Autodesk Fusion 360 part; units mm, degrees
note: some values were not read from the file. Set by a fixed rule: which face or edge a step refers to.
(part 2 of 3)
sketch "Sketch11" plane through (87.5, 0, 0) normal (1, 0, 0) x (0, 1, 0)
  arc A0 (-40.5, 50) -> (-42.5, 48) centre (-40.5, 48) ccw
  line L0 (-42.5, 48) -> (-42.5, 36.5)
  line L1 (-42.5, 36.5) -> (-42, 36.5)
  line L2 (-42, 36.5) -> (-42, 33.5)
  line L3 (-42, 33.5) -> (-42.5, 33.5)
  line L4 (-42.5, 33.5) -> (-42.5, 31.5)
  line L5 (-42.5, 31.5) -> (-42, 31.5)
  line L6 (-42, 31.5) -> (-42, 28.5)
  line L7 (-42, 28.5) -> (-42.5, 28.5)
  line L8 (-42.5, 28.5) -> (-42.5, 26.5)
  line L9 (-42.5, 26.5) -> (-42, 26.5)
  line L10 (-42, 26.5) -> (-42, 23.5)
  line L11 (-42, 23.5) -> (-42.5, 23.5)
  line L12 (-42.5, 23.5) -> (-42.5, 21.5)
  line L13 (-42.5, 21.5) -> (-42, 21.5)
  line L14 (-42, 21.5) -> (-42, 18.5)
  line L15 (-42, 18.5) -> (-42.5, 18.5)
  line L16 (-42.5, 18.5) -> (-42.5, 16.5)
  line L17 (-42.5, 16.5) -> (-42, 16.5)
  line L18 (-42, 16.5) -> (-42, 13.5)
  line L19 (-42, 13.5) -> (-42.5, 13.5)
  line L20 (-42.5, 13.5) -> (-42.5, 2)
  arc A1 (-42.5, 2) -> (-40.5, 0) centre (-40.5, 2) ccw
  line L21 (-40.5, 0) -> (40.5, 0)
  arc A2 (40.5, 0) -> (42.5, 2) centre (40.5, 2) ccw
  line L22 (42.5, 2) -> (42.5, 13.5)
  line L23 (42.5, 13.5) -> (42, 13.5)
  line L24 (42, 13.5) -> (42, 16.5)
  line L25 (42, 16.5) -> (42.5, 16.5)
  line L26 (42.5, 16.5) -> (42.5, 18.5)
  line L27 (42.5, 18.5) -> (42, 18.5)
  line L28 (42, 18.5) -> (42, 21.5)
  line L29 (42, 21.5) -> (42.5, 21.5)
  line L30 (42.5, 21.5) -> (42.5, 23.5)
  line L31 (42.5, 23.5) -> (42, 23.5)
  line L32 (42, 23.5) -> (42, 26.5)
  line L33 (42, 26.5) -> (42.5, 26.5)
  line L34 (42.5, 26.5) -> (42.5, 28.5)
  line L35 (42.5, 28.5) -> (42, 28.5)
  line L36 (42, 28.5) -> (42, 31.5)
  line L37 (42, 31.5) -> (42.5, 31.5)
  line L38 (42.5, 31.5) -> (42.5, 33.5)
  line L39 (42.5, 33.5) -> (42, 33.5)
  line L40 (42, 33.5) -> (42, 36.5)
  line L41 (42, 36.5) -> (42.5, 36.5)
  line L42 (42.5, 36.5) -> (42.5, 48)
  arc A3 (42.5, 48) -> (40.5, 50) centre (40.5, 48) ccw
  line L43 (40.5, 50) -> (34, 50)
  line L44 (34, 50) -> (34, 49.866)
  spline S0 degree 3 poles (33.5, 49) (33.6385, 49.1385) (33.802, 49.3076) (33.9552, 49.5924) (34, 49.7386) (34, 49.866) knots 0 0 0 0 0.058781 0.058781 0.097013 0.097013 0.097013 0.097013
  line L45 (33.5, 49) -> (31.5, 49)
  spline S1 degree 3 poles (31, 49.866) (31, 49.7386) (31.0448, 49.5924) (31.198, 49.3076) (31.3615, 49.1385) (31.5, 49) knots 0.252766 0.252766 0.252766 0.252766 0.290998 0.290998 0.349779 0.349779 0.349779 0.349779
  line L46 (31, 49.866) -> (31, 50)
  line L47 (31, 50) -> (26, 50)
  line L48 (26, 50) -> (26, 49.866)
  spline S2 degree 3 poles (25.5, 49) (25.6385, 49.1385) (25.802, 49.3076) (25.9552, 49.5924) (26, 49.7386) (26, 49.866) knots 0 0 0 0 0.058781 0.058781 0.097013 0.097013 0.097013 0.097013
  line L49 (25.5, 49) -> (23.5, 49)
  spline S3 degree 3 poles (23, 49.866) (23, 49.7386) (23.0448, 49.5924) (23.198, 49.3076) (23.3615, 49.1385) (23.5, 49) knots 0.252766 0.252766 0.252766 0.252766 0.290998 0.290998 0.349779 0.349779 0.349779 0.349779
  line L50 (23, 49.866) -> (23, 50)
  line L51 (23, 50) -> (18, 50)
  line L52 (18, 50) -> (18, 49.866)
  spline S4 degree 3 poles (17.5, 49) (17.6385, 49.1385) (17.802, 49.3076) (17.9552, 49.5924) (18, 49.7386) (18, 49.866) knots 0 0 0 0 0.058781 0.058781 0.097013 0.097013 0.097013 0.097013
  line L53 (17.5, 49) -> (15.5, 49)
  spline S5 degree 3 poles (15, 49.866) (15, 49.7386) (15.0448, 49.5924) (15.198, 49.3076) (15.3615, 49.1385) (15.5, 49) knots 0.252766 0.252766 0.252766 0.252766 0.290998 0.290998 0.349779 0.349779 0.349779 0.349779
  line L54 (15, 49.866) -> (15, 50)
  line L55 (15, 50) -> (-16, 50)
  line L56 (-16, 50) -> (-16, 49.866)
  spline S6 degree 3 poles (-16.5, 49) (-16.3615, 49.1385) (-16.198, 49.3076) (-16.0448, 49.5924) (-16, 49.7386) (-16, 49.866) knots 0 0 0 0 0.058781 0.058781 0.097013 0.097013 0.097013 0.097013
  line L57 (-16.5, 49) -> (-18.5, 49)
  spline S7 degree 3 poles (-19, 49.866) (-19, 49.7386) (-18.9552, 49.5924) (-18.802, 49.3076) (-18.6385, 49.1385) (-18.5, 49) knots 0.252766 0.252766 0.252766 0.252766 0.290998 0.290998 0.349779 0.349779 0.349779 0.349779
  line L58 (-19, 49.866) -> (-19, 50)
  line L59 (-19, 50) -> (-24, 50)
  line L60 (-24, 50) -> (-24, 49.866)
  spline S8 degree 3 poles (-24.5, 49) (-24.3615, 49.1385) (-24.198, 49.3076) (-24.0448, 49.5924) (-24, 49.7386) (-24, 49.866) knots 0 0 0 0 0.058781 0.058781 0.097013 0.097013 0.097013 0.097013
  line L61 (-24.5, 49) -> (-26.5, 49)
  spline S9 degree 3 poles (-27, 49.866) (-27, 49.7386) (-26.9552, 49.5924) (-26.802, 49.3076) (-26.6385, 49.1385) (-26.5, 49) knots 0.252766 0.252766 0.252766 0.252766 0.290998 0.290998 0.349779 0.349779 0.349779 0.349779
  line L62 (-27, 49.866) -> (-27, 50)
  line L63 (-27, 50) -> (-32, 50)
  line L64 (-32, 50) -> (-32, 49.866)
  spline S10 degree 3 poles (-32.5, 49) (-32.3615, 49.1385) (-32.198, 49.3076) (-32.0448, 49.5924) (-32, 49.7386) (-32, 49.866) knots 0 0 0 0 0.058781 0.058781 0.097013 0.097013 0.097013 0.097013
  line L65 (-32.5, 49) -> (-34.5, 49)
  spline S11 degree 3 poles (-35, 49.866) (-35, 49.7386) (-34.9552, 49.5924) (-34.802, 49.3076) (-34.6385, 49.1385) (-34.5, 49) knots 0.252766 0.252766 0.252766 0.252766 0.290998 0.290998 0.349779 0.349779 0.349779 0.349779
  line L66 (-35, 49.866) -> (-35, 50)
  line L67 (-35, 50) -> (-40.5, 50)
  line L68 (-0.5, 50) -> (-0.5, 0) construction
  line L69 (-0.5, 25) -> (-42, 25) construction
  line L70 (-28.75, 32.5) -> (-13.75, 32.5)
  line L71 (-13.75, 32.5) -> (-13.75, 17.5)
  line L72 (-13.75, 17.5) -> (-28.75, 17.5)
  line L73 (-28.75, 17.5) -> (-28.75, 32.5)
  line L74 (-28.75, 32.5) -> (-13.75, 17.5) construction
  line L75 (-13.75, 32.5) -> (-28.75, 17.5) construction
  point P0 (-21.25, 25)
  dimension "d81" = 15
  dimension "d82" = 15
  constraint midpoint L55 L68.start
  constraint coincident L21 L68.end
  constraint perpendicular L21 L68
  constraint midpoint L68 L69.start
  constraint midpoint L10 L69.end
  constraint horizontal L70
  constraint perpendicular L70 L71
  constraint parallel L70 L72
  constraint parallel L71 L73
  constraint coincident L74 P0
  constraint coincident L75 P0
  constraint midpoint L69 P0
  measures "d81" distance of L71.end L72.end
  measures "d82" distance of L70.end L71.end
extrude "Extrude11" add sketch "Sketch11" along normal blind 4 contours L70 L71 L72 L73
sketch "Sketch12" plane through (91.5, 0, 0) normal (1, 0, 0) x (0, 1, 0)
  line L0 (-28.75, 17.5) -> (-13.75, 17.5)
  line L1 (-13.75, 17.5) -> (-13.75, 32.5)
  line L2 (-13.75, 32.5) -> (-28.75, 32.5)
  line L3 (-28.75, 32.5) -> (-28.75, 17.5)
  line L4 (-28.75, 32.5) -> (-13.75, 17.5) construction
  line L5 (-26.25, 30) -> (-16.25, 30)
  line L6 (-16.25, 30) -> (-16.25, 20)
  line L7 (-16.25, 20) -> (-26.25, 20)
  line L8 (-26.25, 20) -> (-26.25, 30)
  line L9 (-26.25, 30) -> (-16.25, 20) construction
  line L10 (-16.25, 30) -> (-26.25, 20) construction
  point P0 (-21.25, 25)
  dimension "d85" = 10
  dimension "d86" = 10
  constraint coincident L2.end L3.start
  constraint coincident L0.end L1.start
  constraint horizontal L5
  constraint perpendicular L5 L6
  constraint parallel L5 L7
  constraint parallel L6 L8
  constraint coincident L9 P0
  constraint coincident L10 P0
  constraint midpoint L4 P0
  measures "d85" distance of L6.end L7.end
  measures "d86" distance of L5.end L6.end
extrude "Extrude12" add sketch "Sketch12" along normal blind 3 contours L5 L6 L7 L8
sketch "Sketch13" plane through (94.5, 0, 0) normal (1, 0, 0) x (0, 1, 0)
  line L0 (-26.25, 20) -> (-16.25, 20)
  line L1 (-16.25, 20) -> (-16.25, 30)
  line L2 (-16.25, 30) -> (-26.25, 30)
  line L3 (-26.25, 30) -> (-26.25, 20)
  line L4 (-26.25, 30) -> (-16.25, 20) construction
  line L5 (-28.75, 32.5) -> (-13.75, 32.5)
  line L6 (-13.75, 32.5) -> (-13.75, 17.5)
  line L7 (-13.75, 17.5) -> (-28.75, 17.5)
  line L8 (-28.75, 17.5) -> (-28.75, 32.5)
  line L9 (-28.75, 32.5) -> (-13.75, 17.5) construction
  line L10 (-13.75, 32.5) -> (-28.75, 17.5) construction
  point P0 (-21.25, 25)
  dimension "d89" = 15
  dimension "d90" = 15
  constraint coincident L2.end L3.start
  constraint coincident L0.end L1.start
  constraint horizontal L5
  constraint perpendicular L5 L6
  constraint parallel L5 L7
  constraint parallel L6 L8
  constraint coincident L9 P0
  constraint coincident L10 P0
  constraint midpoint L4 P0
  measures "d89" distance of L6.end L7.end
  measures "d90" distance of L5.end L6.end
extrude "Extrude13" add sketch "Sketch13" along normal blind 4 contours L0 L1 L2 L3 | L5 L6 L7 L8
sketch "Sketch14" plane through (98.5, 0, 0) normal (1, 0, 0) x (0, 1, 0)
  line L0 (-28.75, 17.5) -> (-13.75, 17.5)
  line L1 (-13.75, 17.5) -> (-13.75, 32.5)
  line L2 (-13.75, 32.5) -> (-28.75, 32.5)
  line L3 (-28.75, 32.5) -> (-28.75, 17.5)
  line L4 (-28.75, 32.5) -> (-13.75, 17.5) construction
  circle A0 centre (-21.25, 25) radius 5
  dimension "d93" = 10
  constraint coincident L2.end L3.start
  constraint coincident L0.end L1.start
  constraint midpoint L4 A0.centre
  measures "d93" diameter of A0
extrude "Extrude14" add sketch "Sketch14" along normal blind 10 contours A0
sketch "Sketch15" plane through (108.5, 0, 0) normal (1, 0, 0) x (0, 1, 0)
  circle A0 centre (-21.25, 25) radius 5
  circle A1 centre (-21.25, 25) radius 4
  dimension "d96" = 8
  constraint concentric A0 A1
  measures "d96" diameter of A1
extrude "Extrude15" add sketch "Sketch15" along normal blind 30 contours A1

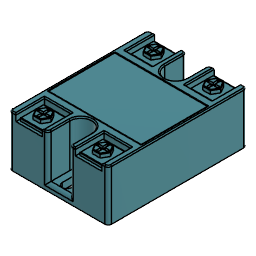
design "SOLID_STATE_Relay"
part number: 2026-09-24-14-23-57-281
Autodesk Fusion 360 part; units mm, degrees
sketch "Sketch1" plane through (0, 0, 0) normal (0, 0, 1) x (1, 0, 0)
  line L0 (0, 0) -> (45, 0)
  line L1 (45, 0) -> (45, 63)
  line L2 (45, 63) -> (0, 63)
  line L3 (0, 63) -> (0, 0)
  dimension "d1" = 45
  dimension "d2" = 63
  constraint horizontal L0
  constraint vertical L1
  constraint horizontal L2
  constraint vertical L3
  constraint coincident L0.start L3.end
  measures "d1" distance of L0.start L0.end
  measures "d2" distance of L0.start L2.end
extrude "Extrude1" add sketch "Sketch1" along normal blind 23.2
sketch "Sketch2" plane through (0, 0, 23.2) normal (0, 0, 1) x (-1, 0, 0)
  line L0 (0, -63) -> (0, 0)
  line L1 (0, 0) -> (-45, 0)
  line L2 (-45, 0) -> (-45, -63)
  line L3 (-45, -63) -> (0, -63)
  line L4 (0, -63) -> (-45, 0) construction
  line L5 (-1.5, -46.5) -> (-43.5, -46.5)
  line L6 (-43.5, -46.5) -> (-43.5, -16.5)
  line L7 (-43.5, -16.5) -> (-1.5, -16.5)
  line L8 (-1.5, -16.5) -> (-1.5, -46.5)
  line L9 (-1.5, -46.5) -> (-43.5, -16.5) construction
  line L10 (-43.5, -46.5) -> (-1.5, -16.5) construction
  point P0 (-22.5, -31.5)
  dimension "d5" = 42
  dimension "d6" = 30
  constraint coincident L0.start L3.end
  constraint coincident L1.end L2.start
  constraint horizontal L5
  constraint perpendicular L5 L6
  constraint parallel L5 L7
  constraint parallel L6 L8
  constraint coincident L9 P0
  constraint coincident L10 P0
  constraint midpoint L4 P0
  measures "d5" distance of L6.end L7.end
  measures "d6" distance of L5.end L6.end
extrude "Extrude2" cut sketch "Sketch2" against normal blind 0.1 contours L5 L6 L7 L8
sketch "Sketch3" plane through (0, 0, 23.2) normal (0, 0, 1) x (-1, 0, 0)
  line L0 (-43.5, -46.5) -> (-43.5, -16.5)
  line L1 (-43.5, -16.5) -> (-1.5, -16.5)
  line L2 (-1.5, -16.5) -> (-1.5, -46.5)
  line L3 (-1.5, -46.5) -> (-43.5, -46.5)
  line L4 (0, -63) -> (0, 0)
  line L5 (0, 0) -> (-45, 0)
  line L6 (-45, 0) -> (-45, -63)
  line L7 (-45, -63) -> (0, -63)
  line L8 (-3.1245, -63) -> (-15.1245, -63)
  line L9 (-15.1245, -63) -> (-15.1245, -50)
  line L10 (-15.1245, -50) -> (-3.1245, -50)
  line L11 (-3.1245, -50) -> (-3.1245, -63)
  dimension "d9" = 12
  constraint horizontal L8
  constraint vertical L9
  constraint horizontal L10
  constraint vertical L11
  constraint coincident L7 L8.start
  measures "d9" distance of L8.start L8.end
extrude "Extrude3" cut sketch "Sketch3" against normal blind 3 contours L7 L8 L9 L10 L11
pattern_linear "R-Pattern1" count 2 spacing 50 along (0, -1, 0) count 2 spacing 27 along (1, 0, 0) of "Extrude3"
sketch "Sketch4" plane through (0, 0, 20.2) normal (0, 0, 1) x (-1, 0, 0)
  line L0 (-3.1245, -50) -> (-15.1245, -50)
  line L1 (-15.1245, -50) -> (-15.1245, -63)
  line L2 (-15.1245, -63) -> (-3.1245, -63)
  line L3 (-3.1245, -63) -> (-3.1245, -50)
  line L4 (-3.1245, -63) -> (-15.1245, -50) construction
  line L5 (-3.8745, -61.75) -> (-14.3745, -61.75)
  line L6 (-14.3745, -61.75) -> (-14.3745, -51.25)
  line L7 (-14.3745, -51.25) -> (-3.8745, -51.25)
  line L8 (-3.8745, -51.25) -> (-3.8745, -61.75)
  line L9 (-3.8745, -61.75) -> (-14.3745, -51.25) construction
  line L10 (-14.3745, -61.75) -> (-3.8745, -51.25) construction
  point P0 (-9.1245, -56.5)
  dimension "d16" = 10.5
  dimension "d17" = 10.5
  constraint coincident L2.end L3.start
  constraint coincident L0.end L1.start
  constraint horizontal L5
  constraint perpendicular L5 L6
  constraint parallel L5 L7
  constraint parallel L6 L8
  constraint coincident L9 P0
  constraint coincident L10 P0
  constraint midpoint L4 P0
  measures "d16" distance of L6.end L7.end
  measures "d17" distance of L5.end L6.end
extrude "Extrude4" add sketch "Sketch4" along normal blind 1.25 contours L5 L6 L7 L8
sketch "Sketch5" plane through (0, 0, 21.45) normal (0, 0, 1) x (-1, 0, 0)
  line L0 (-3.8745, -51.25) -> (-14.3745, -51.25)
  line L1 (-14.3745, -51.25) -> (-14.3745, -61.75)
  line L2 (-14.3745, -61.75) -> (-3.8745, -61.75)
  line L3 (-3.8745, -61.75) -> (-3.8745, -51.25)
  line L4 (-14.3745, -51.25) -> (-3.8745, -61.75) construction
  line L5 (-10.8423, -53.4918) -> (-12.5886, -56.4836)
  line L6 (-12.5886, -56.4836) -> (-10.8708, -59.4918)
  line L7 (-10.8708, -59.4918) -> (-7.4067, -59.5082)
  line L8 (-7.4067, -59.5082) -> (-5.6605, -56.5164)
  line L9 (-5.6605, -56.5164) -> (-7.3783, -53.5082)
  line L10 (-7.3783, -53.5082) -> (-10.8423, -53.4918)
  point P0 (-9.1245, -56.5)
  dimension "d20" = 3
  constraint coincident L0.end L1.start
  constraint coincident L2.end L3.start
  constraint midpoint L4 P0
  measures "d20" distance of P0 L10
extrude "Extrude5" add sketch "Sketch5" along normal blind 1.75 contours L5 L6 L7 L8 L9 L10
sketch "Sketch6" plane through (0, 0, 23.2) normal (0, 0, 1) x (-1, 0, 0)
  line L0 (-7.3783, -53.5082) -> (-10.8423, -53.4918)
  line L1 (-10.8423, -53.4918) -> (-12.5886, -56.4836)
  line L2 (-12.5886, -56.4836) -> (-10.8708, -59.4918)
  line L3 (-10.8708, -59.4918) -> (-7.4067, -59.5082)
  line L4 (-7.4067, -59.5082) -> (-5.6605, -56.5164)
  line L5 (-5.6605, -56.5164) -> (-7.3783, -53.5082)
  line L6 (-9.1103, -53.5) -> (-9.1388, -59.5) construction
  line L7 (-11.6245, -56) -> (-6.6245, -56)
  line L8 (-6.6245, -56) -> (-6.6245, -57)
  line L9 (-6.6245, -57) -> (-11.6245, -57)
  line L10 (-11.6245, -57) -> (-11.6245, -56)
  line L11 (-11.6245, -56) -> (-6.6245, -57) construction
  line L12 (-6.6245, -56) -> (-11.6245, -57) construction
  line L13 (-9.6245, -54) -> (-8.6245, -54)
  line L14 (-8.6245, -54) -> (-8.6245, -59)
  line L15 (-8.6245, -59) -> (-9.6245, -59)
  line L16 (-9.6245, -59) -> (-9.6245, -54)
  line L17 (-9.6245, -54) -> (-8.6245, -59) construction
  line L18 (-8.6245, -54) -> (-9.6245, -59) construction
  point P0 (-9.1245, -56.5)
  point P1 (-9.1245, -56.5)
  dimension "d23" = 5
  dimension "d24" = 1
  dimension "d25" = 1
  dimension "d26" = 5
  constraint midpoint L0 L6.start
  constraint midpoint L3 L6.end
  constraint horizontal L7
  constraint perpendicular L7 L8
  constraint parallel L7 L9
  constraint parallel L8 L10
  constraint coincident L11 P1
  constraint coincident L12 P1
  constraint midpoint L6 P1
  constraint horizontal L13
  constraint perpendicular L13 L14
  constraint parallel L13 L15
  constraint parallel L14 L16
  constraint coincident L17 P1
  constraint coincident L18 P1
  constraint coincident P1 P0
  measures "d23" distance of L8.end L9.end
  measures "d24" distance of L7.end L8.end
  measures "d25" distance of L14.end L15.end
  measures "d26" distance of L13.end L14.end
extrude "Extrude6" cut sketch "Sketch6" against normal blind 1 contours L7 L9 L10 L16 | L7 L13 L14 L16 | L7 L9 L14 L16 | L7 L8 L9 L14 | L9 L14 L15 L16
fillet "Fillet1" radius 0.25 6 edges at (6.5336, 58.0123, 23.2) (9.1388, 59.5, 23.2) (11.7297, 57.9877, 23.2) (11.7155, 54.9877, 23.2) (9.1103, 53.5, 23.2) (6.5194, 55.0123, 23.2)
fillet "Fillet2" radius 0.2 4 edges at (9.1245, 51.25, 21.45) (3.8745, 56.5, 21.45) (9.1245, 61.75, 21.45) (14.3745, 56.5, 21.45)
pattern_linear "R-Pattern2" count 2 spacing 50 along (0, -1, 0) count 2 spacing 27 along (1, 0, 0) of "Extrude4", "Extrude5", "Extrude6", "Fillet1", "Fillet2"
fillet "Fillet3" radius 1.5 4 edges at (0, 63, 11.6) (45, 63, 11.6) (0, 0, 11.6) (45, 0, 11.6)
sketch "Sketch7" plane through (0, 0, 23.2) normal (0, 0, 1) x (-1, 0, 0)
  arc A0 (-43.5, 0) -> (-45, -1.5) centre (-43.5, -1.5) ccw
  line L0 (-45, -1.5) -> (-45, -61.5)
  arc A1 (-45, -61.5) -> (-43.5, -63) centre (-43.5, -61.5) ccw
  line L1 (-43.5, -63) -> (-42.1245, -63)
  line L2 (-42.1245, -63) -> (-42.1245, -50)
  line L3 (-42.1245, -50) -> (-30.1245, -50)
  line L4 (-30.1245, -50) -> (-30.1245, -63)
  line L5 (-30.1245, -63) -> (-15.1245, -63)
  line L6 (-15.1245, -63) -> (-15.1245, -50)
  line L7 (-15.1245, -50) -> (-3.1245, -50)
  line L8 (-3.1245, -50) -> (-3.1245, -63)
  line L9 (-3.1245, -63) -> (-1.5, -63)
  arc A2 (-1.5, -63) -> (0, -61.5) centre (-1.5, -61.5) ccw
  line L10 (0, -61.5) -> (0, -1.5)
  arc A3 (0, -1.5) -> (-1.5, 0) centre (-1.5, -1.5) ccw
  line L11 (-1.5, 0) -> (-3.1245, 0)
  line L12 (-3.1245, 0) -> (-3.1245, -13)
  line L13 (-3.1245, -13) -> (-15.1245, -13)
  line L14 (-15.1245, -13) -> (-15.1245, 0)
  line L15 (-15.1245, 0) -> (-30.1245, 0)
  line L16 (-30.1245, 0) -> (-30.1245, -13)
  line L17 (-30.1245, -13) -> (-42.1245, -13)
  line L18 (-42.1245, -13) -> (-42.1245, 0)
  line L19 (-42.1245, 0) -> (-43.5, 0)
  line L20 (-43.5, -46.5) -> (-43.5, -16.5)
  line L21 (-43.5, -16.5) -> (-1.5, -16.5)
  line L22 (-1.5, -16.5) -> (-1.5, -46.5)
  line L23 (-1.5, -46.5) -> (-43.5, -46.5)
  line L24 (-27.6245, 10) -> (-27.6245, -10)
  arc A4 (-27.6245, -10) -> (-17.6245, -10) centre (-22.6245, -10) ccw
  line L25 (-17.6245, -10) -> (-17.6245, 10)
  arc A5 (-17.6245, 10) -> (-27.6245, 10) centre (-22.6245, 10) ccw
  line L26 (-22.6245, 10) -> (-22.6245, -10) construction
  point P0 (-22.6245, 0)
  dimension "d39" = 10
  constraint tangent L24 A4
  constraint tangent A4 L25
  constraint parallel L24 L25
  constraint tangent L25 A5
  constraint tangent L24 A5
  constraint perpendicular L15 L26
  constraint midpoint L15 P0
  constraint midpoint L26 P0
  measures "d39" diameter of A4
extrude "Extrude7" cut sketch "Sketch7" against normal blind 20 contours L15 L24 A4 L25
fillet "Fillet4" radius 1.5 3 edges at (27.6245, 0, 13.2) (17.6245, 0, 13.2) (22.6245, 0, 3.2)
sketch "Sketch8" plane through (0, 0, 3.2) normal (0, 0, 1) x (-1, 0, 0)
  line L0 (-27.6245, -1.5) -> (-27.6245, -10)
  arc A0 (-27.6245, -10) -> (-17.6245, -10) centre (-22.6245, -10) ccw
  line L1 (-17.6245, -10) -> (-17.6245, -1.5)
  line L2 (-22.6245, -15) -> (-22.6245, 0) construction
  line L3 (-24.6245, -3.5) -> (-24.6245, -11.5)
  arc A1 (-24.6245, -11.5) -> (-20.6245, -11.5) centre (-22.6245, -11.5) ccw
  line L4 (-20.6245, -11.5) -> (-20.6245, -3.5)
  arc A2 (-20.6245, -3.5) -> (-24.6245, -3.5) centre (-22.6245, -3.5) ccw
  line L5 (-22.6245, -3.5) -> (-22.6245, -11.5) construction
  line L6 (-17.6245, -1.5) -> (-27.6245, -1.5)
  point P0 (-22.6245, -7.5)
  dimension "d44" = 4
  constraint midpoint A0 L2.start
  constraint tangent L3 A1
  constraint tangent A1 L4
  constraint parallel L3 L4
  constraint tangent L4 A2
  constraint tangent L3 A2
  constraint midpoint L2 P0
  constraint midpoint L5 P0
  measures "d44" diameter of A1
extrude "Extrude8" cut sketch "Sketch8" against normal blind 3.2 contours L3 A1 L4 A2
sketch "Sketch9" plane through (0, 0, 23.2) normal (0, 0, 1) x (-1, 0, 0)
  line L0 (-43.5, -46.5) -> (-43.5, -16.5)
  line L1 (-43.5, -16.5) -> (-1.5, -16.5)
  line L2 (-1.5, -16.5) -> (-1.5, -46.5)
  line L3 (-1.5, -46.5) -> (-43.5, -46.5)
  arc A0 (-16.1245, 0) -> (-17.6245, -1.5) centre (-16.1245, -1.5) ccw
  line L4 (-17.6245, -1.5) -> (-17.6245, -10)
  arc A1 (-27.6245, -10) -> (-17.6245, -10) centre (-22.6245, -10) ccw
  line L5 (-27.6245, -10) -> (-27.6245, -1.5)
  arc A2 (-27.6245, -1.5) -> (-29.1245, 0) centre (-29.1245, -1.5) ccw
  line L6 (-29.1245, 0) -> (-30.1245, 0)
  line L7 (-30.1245, 0) -> (-30.1245, -13)
  line L8 (-30.1245, -13) -> (-42.1245, -13)
  line L9 (-42.1245, -13) -> (-42.1245, 0)
  line L10 (-42.1245, 0) -> (-43.5, 0)
  arc A3 (-43.5, 0) -> (-45, -1.5) centre (-43.5, -1.5) ccw
  line L11 (-45, -1.5) -> (-45, -61.5)
  arc A4 (-45, -61.5) -> (-43.5, -63) centre (-43.5, -61.5) ccw
  line L12 (-43.5, -63) -> (-42.1245, -63)
  line L13 (-42.1245, -63) -> (-42.1245, -50)
  line L14 (-42.1245, -50) -> (-30.1245, -50)
  line L15 (-30.1245, -50) -> (-30.1245, -63)
  line L16 (-30.1245, -63) -> (-15.1245, -63)
  line L17 (-15.1245, -63) -> (-15.1245, -50)
  line L18 (-15.1245, -50) -> (-3.1245, -50)
  line L19 (-3.1245, -50) -> (-3.1245, -63)
  line L20 (-3.1245, -63) -> (-1.5, -63)
  arc A5 (-1.5, -63) -> (0, -61.5) centre (-1.5, -61.5) ccw
  line L21 (0, -61.5) -> (0, -1.5)
  arc A6 (0, -1.5) -> (-1.5, 0) centre (-1.5, -1.5) ccw
  line L22 (-1.5, 0) -> (-3.1245, 0)
  line L23 (-3.1245, 0) -> (-3.1245, -13)
  line L24 (-3.1245, -13) -> (-15.1245, -13)
  line L25 (-15.1245, -13) -> (-15.1245, 0)
  line L26 (-15.1245, 0) -> (-16.1245, 0)
  line L27 (-17.6245, -73) -> (-17.6245, -53)
  arc A7 (-17.6245, -53) -> (-27.6245, -53) centre (-22.6245, -53) ccw
  line L28 (-27.6245, -53) -> (-27.6245, -73)
  arc A8 (-27.6245, -73) -> (-17.6245, -73) centre (-22.6245, -73) ccw
  line L29 (-22.6245, -73) -> (-22.6245, -53) construction
  point P0 (-22.6245, -63)
  dimension "d47" = 10
  dimension "d48" = 10
  constraint tangent L27 A7
  constraint tangent A7 L28
  constraint parallel L27 L28
  constraint tangent L28 A8
  constraint tangent L27 A8
  constraint perpendicular L16 L29
  constraint midpoint L16 P0
  constraint midpoint L29 P0
  measures "d47" distance of A7.centre P0
  measures "d48" diameter of A7
extrude "Extrude9" cut sketch "Sketch9" against normal blind 20 contours L16 L27 A7 L28
sketch "Sketch10" plane through (0, 0, 3.2) normal (0, 0, 1) x (-1, 0, 0)
  line L0 (-27.6245, -53) -> (-27.6245, -63)
  line L1 (-27.6245, -63) -> (-17.6245, -63)
  line L2 (-17.6245, -63) -> (-17.6245, -53)
  arc A0 (-17.6245, -53) -> (-27.6245, -53) centre (-22.6245, -53) ccw
  line L3 (-22.6245, -48) -> (-22.6245, -63) construction
  line L4 (-20.6245, -59.5) -> (-20.6245, -51.5)
  arc A1 (-20.6245, -51.5) -> (-24.6245, -51.5) centre (-22.6245, -51.5) ccw
  line L5 (-24.6245, -51.5) -> (-24.6245, -59.5)
  arc A2 (-24.6245, -59.5) -> (-20.6245, -59.5) centre (-22.6245, -59.5) ccw
  line L6 (-22.6245, -59.5) -> (-22.6245, -51.5) construction
  point P0 (-22.6245, -55.5)
  dimension "d51" = 4
  constraint midpoint A0 L3.start
  constraint midpoint L1 L3.end
  constraint tangent L4 A1
  constraint tangent A1 L5
  constraint parallel L4 L5
  constraint tangent L5 A2
  constraint tangent L4 A2
  constraint parallel L3 L6
  constraint midpoint L3 P0
  constraint midpoint L6 P0
  measures "d51" diameter of A1
extrude "Extrude10" cut sketch "Sketch10" against normal blind 3.2 contours L4 A1 L5 A2
fillet "Fillet5" radius 1.5 3 edges at (17.6245, 63, 13.2) (22.6245, 63, 3.2) (27.6245, 63, 13.2)
fillet "Fillet6" radius 0.5 1 faces at (2.083, 4.8333, 23.2)

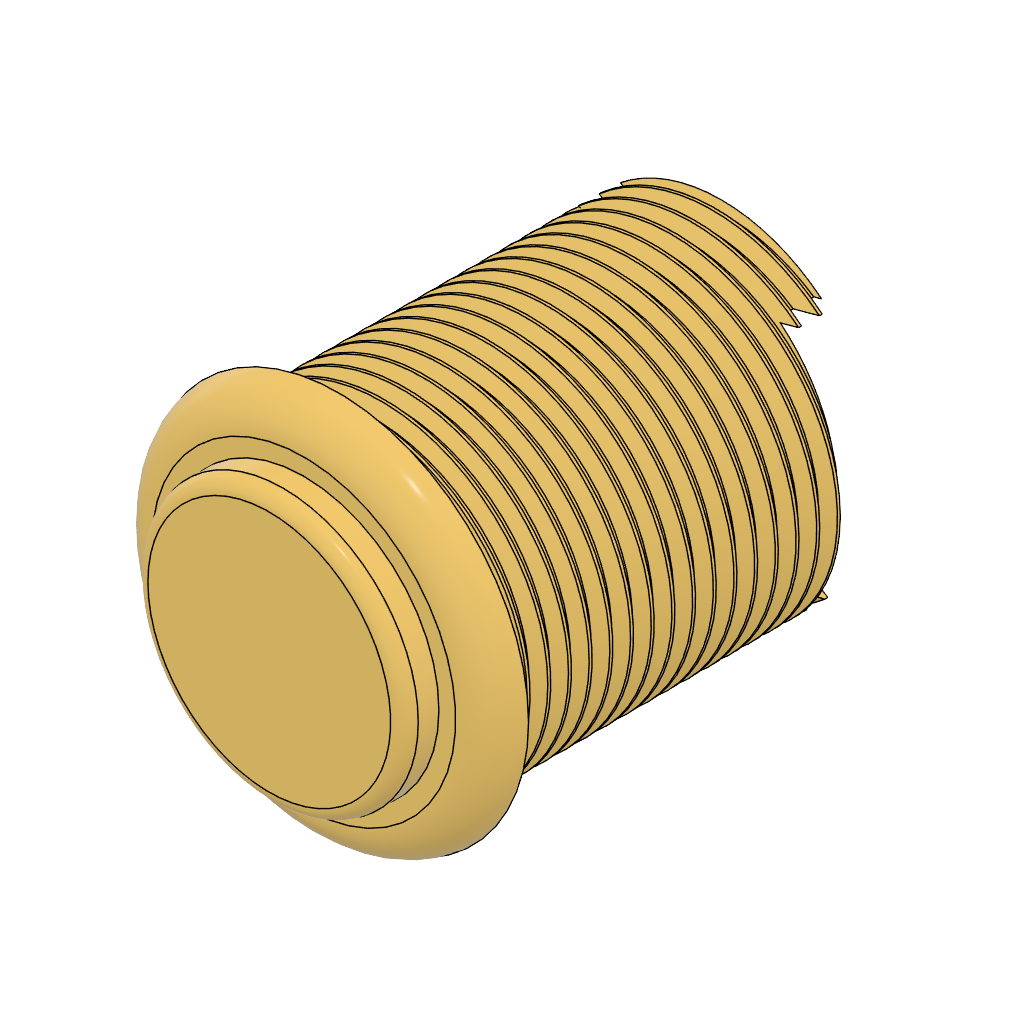
design "ArcadeButton"
part number: 2026-09-25-10-11-44-145
Autodesk Fusion 360 part; units mm, degrees
sketch "Sketch1" plane through (0, 0, 0) normal (0, 0, 1) x (1, 0, 0)
  circle A0 centre (0, 0) radius 9.8
  dimension "d1" = 19.6
  constraint coincident A0.centre origin
  measures "d1" diameter of A0
extrude "Extrude1" add sketch "Sketch1" along normal blind 2.5 makes body 1
fillet "Fillet1" radius 1 1 edges at (-9.1368, -3.5438, 2.5) on bodies 1
sketch "Sketch2" plane through (0, 0, 0) normal (0, 0, -1) x (-1, 0, 0)
  circle A0 centre (0, 0) radius 9.8
  circle A1 centre (0, 0) radius 13.8
  dimension "d6" = 27.6
  constraint concentric A0 A1
  measures "d6" diameter of A1
extrude "Extrude2" add sketch "Sketch2" along normal blind 2.5 separate body makes body 2
fillet "Fillet2" radius 2.8 1 edges at (12.8661, -4.9903, 0) on bodies 2
sketch "Sketch3" plane through (0, 0, -2.5) normal (0, 0, -1) x (-1, 0, 0)
  circle A0 centre (0, 0) radius 9.8
  circle A1 centre (0, 0) radius 13.8
  circle A2 centre (0, 0) radius 12
  dimension "d11" = 24
  constraint coincident A0.centre A1.centre
  measures "d11" diameter of A2
extrude "Extrude3" add sketch "Sketch3" along normal blind 28.2 contours A2 bodies 2
thread "Thread1" "ISO Metric profile 24.0 M24x1.5 M24x1.5 6g" major diameter 23.85 minor diameter 22.1319 pitch 1.5 angle 60 modelled right hand crest width 0.2123 on face at (-11.9851, -0.5982, -21.3) crest through (-11.925, 0, -2.125) on bodies 2
sketch "Sketch4" plane through (0, 0, 0) normal (0, 0, -1) x (-1, 0, 0)
  circle A0 centre (0, 0) radius 9.8
extrude "Extrude4" add sketch "Sketch4" along normal blind 30.7 bodies 1 2
sketch "Sketch5" plane through (0, 0, -30.7) normal (0, 0, -1) x (-1, 0, 0)
  spline S0 degree 3 poles (-6.584, -8.8942) (-5.4514, -9.7999) (-4.1518, -10.4742) (-1.348, -11.2962) (0.1314, -11.4284) (3.0791, -11.12) (4.5181, -10.6746) (7.1649, -9.2503) (8.3434, -8.2785) (9.955, -6.3167) (10.4989, -5.4424) (11.3511, -3.5668) (11.6534, -2.5726) (11.8236, -1.5519) knots 0 0 0 0 0.435068 0.435068 0.876287 0.876287 1.323654 1.323654 1.777168 1.777168 2.08439 2.08439 2.394399 2.394399 2.394399 2.394399
  arc A0 (11.8236, -1.5519) -> (8.6533, 8.2053) centre (0, 0) ccw
  spline S1 degree 3 poles (8.6533, 8.2053) (7.5544, 9.2865) (6.2561, 10.1443) (3.4216, 11.3024) (1.9157, 11.599) (-1.1044, 11.5943) (-2.5895, 11.301) (-5.3429, 10.1661) (-6.5878, 9.3427) (-8.3338, 7.6141) (-8.9365, 6.838) (-9.9197, 5.1568) (-10.2979, 4.2601) (-10.5544, 3.3256) knots 0 0 0 0 0.462513 0.462513 0.918871 0.918871 1.369074 1.369074 1.813119 1.813119 2.107031 2.107031 2.398149 2.398149 2.398149 2.398149
  arc A1 (-10.5544, 3.3256) -> (-6.584, -8.8942) centre (0, 0) ccw
  line L0 (-20.0682, 9) -> (20.0682, 9)
  line L1 (20.0682, 9) -> (20.0682, -9)
  line L2 (20.0682, -9) -> (-20.0682, -9)
  line L3 (-20.0682, -9) -> (-20.0682, 9)
  line L4 (-20.0682, 9) -> (20.0682, -9) construction
  line L5 (20.0682, 9) -> (-20.0682, -9) construction
  dimension "d18" = 18
  constraint horizontal L0
  constraint perpendicular L0 L1
  constraint parallel L0 L2
  constraint parallel L1 L3
  constraint coincident L4 A0.centre
  constraint coincident L5 A0.centre
  constraint coincident A0.centre A1.centre
  measures "d18" distance of L0.end L1.end
extrude "Extrude5" cut sketch "Sketch5" against normal blind 3 contours S0 A0 S1 A1 L0 L2 | S0 S1 A1 L0 L2 L3 | S0 A0 S1 L0 L1 L2 bodies 1
sketch "Sketch6" plane through (0, 0, -27.7) normal (0, 0, -1) x (-1, 0, 0)
  spline S0 degree 3 poles (-10.5544, 3.3256) (-10.2161, 4.5582) (-9.6666, 5.7229) (-8.3471, 7.6043) (-7.6513, 8.354) (-6.8657, 9) knots -0.772094 -0.772094 -0.772094 -0.772094 -0.388447 -0.388447 -0.082557 -0.082557 -0.082557 -0.082557
  arc A0 (-10.5544, 3.3256) -> (-6.584, -8.8942) centre (0, 0) ccw
  spline S1 degree 3 poles (-6.4495, -9) (-6.4946, -8.9651) (-6.5395, -8.9298) (-6.584, -8.8942) knots -0.017113 -0.017113 -0.017113 -0.017113 0 0 0 0
  line L0 (-6.4495, -9) -> (7.3379, -9)
  spline S2 degree 3 poles (11.8236, -1.5519) (11.6793, -2.4175) (11.4399, -3.2645) (10.7806, -4.8837) (10.3641, -5.6514) (9.1657, -7.3727) (8.3124, -8.2616) (7.3379, -9) knots -0.97951 -0.97951 -0.97951 -0.97951 -0.716355 -0.716355 -0.455211 -0.455211 -0.087339 -0.087339 -0.087339 -0.087339
  arc A1 (11.8236, -1.5519) -> (8.6533, 8.2053) centre (0, 0) ccw
  spline S3 degree 3 poles (7.76, 9) (8.0707, 8.7503) (8.3689, 8.4851) (8.6533, 8.2053) knots -0.119698 -0.119698 -0.119698 -0.119698 0 0 0 0
  line L1 (7.76, 9) -> (-6.8657, 9)
  line L2 (-5, 5) -> (5, 5) construction
  line L3 (5, 5) -> (5, -5) construction
  line L4 (5, -5) -> (-5, -5) construction
  line L5 (-5, -5) -> (-5, 5) construction
  line L6 (-5, 5) -> (5, -5) construction
  line L7 (5, 5) -> (-5, -5) construction
  line L8 (-1.4, 5.5) -> (1.4, 5.5)
  line L9 (1.4, 5.5) -> (1.4, 4.5)
  line L10 (1.4, 4.5) -> (-1.4, 4.5)
  line L11 (-1.4, 4.5) -> (-1.4, 5.5)
  line L12 (-1.4, 5.5) -> (1.4, 4.5) construction
  line L13 (1.4, 5.5) -> (-1.4, 4.5) construction
  line L14 (-1.4, -4.5) -> (1.4, -4.5)
  line L15 (1.4, -4.5) -> (1.4, -5.5)
  line L16 (1.4, -5.5) -> (-1.4, -5.5)
  line L17 (-1.4, -5.5) -> (-1.4, -4.5)
  line L18 (-1.4, -4.5) -> (1.4, -5.5) construction
  line L19 (1.4, -4.5) -> (-1.4, -5.5) construction
  point P0 (0, 5)
  point P1 (0, -5)
  dimension "d21" = 10
  dimension "d22" = 10
  dimension "d23" = 2.8
  dimension "d24" = 1
  dimension "d25" = 2.8
  dimension "d26" = 1
  constraint horizontal L2
  constraint perpendicular L2 L3
  constraint parallel L2 L4
  constraint parallel L3 L5
  constraint coincident L6 A0.centre
  constraint coincident L7 A0.centre
  constraint coincident A0.centre A1.centre
  constraint horizontal L8
  constraint perpendicular L8 L9
  constraint parallel L8 L10
  constraint parallel L9 L11
  constraint coincident L12 P0
  constraint coincident L13 P0
  constraint midpoint L2 P0
  constraint horizontal L14
  constraint perpendicular L14 L15
  constraint parallel L14 L16
  constraint parallel L15 L17
  constraint coincident L18 P1
  constraint coincident L19 P1
  constraint midpoint L4 P1
  measures "d21" distance of L3.end L4.end
  measures "d22" distance of L2.end L3.end
  measures "d23" distance of L9.end L10.end
  measures "d24" distance of L8.end L9.end
  measures "d25" distance of L15.end L16.end
  measures "d26" distance of L14.end L15.end
extrude "Extrude6" add sketch "Sketch6" along normal blind 5 contours L8 L9 L10 L11 | L14 L15 L16 L17 bodies 1
fillet "Fillet3" radius 0.5 4 edges at (1.4, 5, -32.7) (-1.4, 5, -32.7) (-1.4, -5, -32.7) (1.4, -5, -32.7) on bodies 1
sketch "Sketch7" plane through (0, -5.5, 0) normal (0, -1, 0) x (1, 0, 0)
  arc A0 (0.9, -32.7) -> (1.4, -32.2) centre (0.9, -32.2) ccw
  line L0 (1.4, -32.2) -> (1.4, -27.7)
  line L1 (1.4, -27.7) -> (-1.4, -27.7)
  line L2 (-1.4, -27.7) -> (-1.4, -32.2)
  arc A1 (-1.4, -32.2) -> (-0.9, -32.7) centre (-0.9, -32.2) ccw
  line L3 (-0.9, -32.7) -> (0.9, -32.7)
  line L4 (1.4, -31.1987) -> (-1.4, -31.1987) construction
  circle A2 centre (0, -31.1987) radius 0.5
  dimension "d31" = 1
  constraint coincident L0 L4.start
  constraint coincident L2 L4.end
  constraint perpendicular L2 L4
  constraint midpoint L4 A2.centre
  measures "d31" diameter of A2
extrude "Extrude7" cut sketch "Sketch7" against normal blind 11 contours A2 bodies 1
sketch "Sketch8" plane through (0, 0, -30.7) normal (0, 0, -1) x (-1, 0, 0)
  line L0 (-6.8657, 9) -> (7.76, 9)
  spline S0 degree 3 poles (7.76, 9) (6.8728, 9.7127) (5.8864, 10.2953) (3.4216, 11.3024) (1.9157, 11.599) (-1.1044, 11.5943) (-2.5895, 11.301) (-5.0213, 10.2987) (-5.9954, 9.7157) (-6.8657, 9) knots 0.119865 0.119865 0.119865 0.119865 0.462513 0.462513 0.918871 0.918871 1.369074 1.369074 1.708669 1.708669 1.708669 1.708669
  circle A0 centre (0, 0) radius 10.75
  line L1 (-4.8923, -7.1081) -> (4.8923, -7.1081)
  line L2 (4.8923, -7.1081) -> (4.8923, 7.1081)
  line L3 (4.8923, 7.1081) -> (-4.8923, 7.1081)
  line L4 (-4.8923, 7.1081) -> (-4.8923, -7.1081)
  line L5 (-4.8923, -7.1081) -> (4.8923, 7.1081) construction
  line L6 (4.8923, -7.1081) -> (-4.8923, 7.1081) construction
  dimension "d34" = 21.5
  constraint coincident A0.centre origin
  constraint horizontal L1
  constraint perpendicular L1 L2
  constraint parallel L1 L3
  constraint parallel L2 L4
  constraint coincident L5 A0.centre
  constraint coincident L6 A0.centre
  measures "d34" diameter of A0
extrude "Extrude8" cut sketch "Sketch8" against normal blind 3 contours L0 A0 | L0 A0 bodies 1

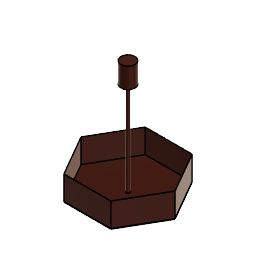
design "Umbrella"
part number: 2026-09-24-17-24-27-584
Autodesk Fusion 360 part; units mm, degrees
sketch "Sketch1" plane through (0, 0, 0) normal (0, 0, 1) x (1, 0, 0)
  line L0 (-57.735, 100) -> (-115.4701, 0)
  line L1 (-115.4701, 0) -> (-57.735, -100)
  line L2 (-57.735, -100) -> (57.735, -100)
  line L3 (57.735, -100) -> (115.4701, 0)
  line L4 (115.4701, 0) -> (57.735, 100)
  line L5 (57.735, 100) -> (-57.735, 100)
  dimension "d1" = 100
  measures "d1" distance of origin L5
extrude "Extrude1" add sketch "Sketch1" along normal blind 60
shell "Shell1" thickness 0.2 removed faces 1 at (19.245, 33.3333, 60)
sketch "Sketch2" plane through (0, 0, 0.2) normal (0, 0, 1) x (-1, 0, 0)
  line L0 (-57.6196, -99.8) -> (57.6196, -99.8)
  line L1 (57.6196, -99.8) -> (115.2391, 0)
  line L2 (115.2391, 0) -> (57.6196, 99.8)
  line L3 (57.6196, 99.8) -> (-57.6196, 99.8)
  line L4 (-57.6196, 99.8) -> (-115.2391, 0)
  line L5 (-115.2391, 0) -> (-57.6196, -99.8)
  circle A0 centre (0, 0) radius 4
  dimension "d5" = 8
  constraint coincident A0.centre origin
  measures "d5" diameter of A0
extrude "Extrude2" add sketch "Sketch2" along normal blind 280 contours A0
sketch "Sketch3" plane through (0, 0, 280.2) normal (0, 0, 1) x (-1, 0, 0)
  circle A0 centre (0, 0) radius 4
  circle A1 centre (0, 0) radius 17.5
  dimension "d8" = 35
  constraint coincident A0.centre A1.centre
  measures "d8" diameter of A1
extrude "Extrude3" add sketch "Sketch3" against normal blind 50
extrude "Extrude4" add 1 faces at (-58.7212, 34.0178, 0.2) along direction (0, 0, 1) blind 1
sketch "Sketch4" plane through (0, 0, 0) normal (0, 0, -1) x (1, 0, 0)
  line L0 (-57.735, -100) -> (57.735, -100)
  line L1 (57.735, -100) -> (115.4701, 0)
  line L2 (115.4701, 0) -> (57.735, 100)
  line L3 (57.735, 100) -> (-57.735, 100)
  line L4 (-57.735, 100) -> (-115.4701, 0)
  line L5 (-115.4701, 0) -> (-57.735, -100)
  circle A0 centre (0, 0) radius 5
  dimension "d13" = 10
  constraint coincident A0.centre origin
  measures "d13" diameter of A0
extrude "Extrude5" add sketch "Sketch4" along normal blind 7 contours A0
chamfer "Chamfer1" distance 1 distance2 7 1 edges at (-4.6616, 1.8081, -7) measured on face at (1.3101, 1.9935, -7)
sketch "Sketch5" plane through (0, 0, 0) normal (0, 0, 1) x (1, 0, 0)

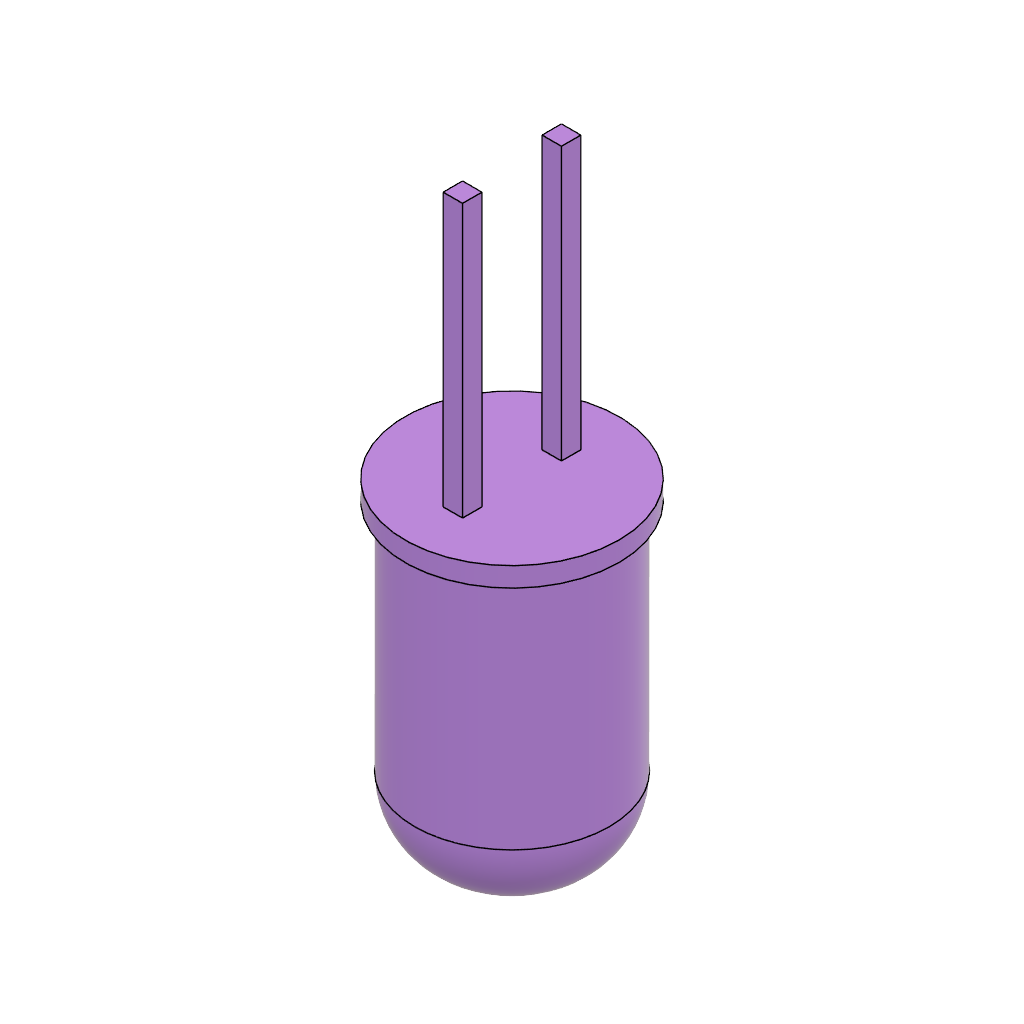
design "Led"
part number: 2026-09-25-11-08-29-165
Autodesk Fusion 360 part; units mm, degrees
sketch "Sketch1" plane through (0, 0, 0) normal (0, 1, 0) x (1, 0, 0)
  circle A0 centre (0, 0) radius 2.5
  dimension "d1" = 5
  constraint coincident A0.centre origin
  measures "d1" diameter of A0
extrude "Extrude1" add sketch "Sketch1" along normal blind 8.5
fillet "Fillet1" radius 2 1 edges at (-2.3308, 0, 0.904)
sketch "Sketch2" plane through (0, 8.5, 0) normal (0, 1, 0) x (-1, 0, 0)
  circle A0 centre (0, 0) radius 2.5
  circle A1 centre (0, 0) radius 2.75
  dimension "d6" = 5.5
  constraint coincident A0.centre A1.centre
  measures "d6" diameter of A1
extrude "Extrude2" add sketch "Sketch2" against normal blind 0.5
sketch "Sketch3" plane through (0, 8.5, 0) normal (0, 1, 0) x (-1, 0, 0)
  circle A0 centre (0, 0) radius 2.75
  line L0 (-1.27, 1.27) -> (1.27, 1.27) construction
  line L1 (1.27, 1.27) -> (1.27, -1.27) construction
  line L2 (1.27, -1.27) -> (-1.27, -1.27) construction
  line L3 (-1.27, -1.27) -> (-1.27, 1.27) construction
  line L4 (-1.27, 1.27) -> (1.27, -1.27) construction
  line L5 (1.27, 1.27) -> (-1.27, -1.27) construction
  line L6 (0.25, 1.02) -> (-0.25, 1.02)
  line L7 (-0.25, 1.02) -> (-0.25, 1.52)
  line L8 (-0.25, 1.52) -> (0.25, 1.52)
  line L9 (0.25, 1.52) -> (0.25, 1.02)
  line L10 (0.25, 1.02) -> (-0.25, 1.52) construction
  line L11 (-0.25, 1.02) -> (0.25, 1.52) construction
  line L12 (-0.25, -1.02) -> (0.25, -1.02)
  line L13 (0.25, -1.02) -> (0.25, -1.52)
  line L14 (0.25, -1.52) -> (-0.25, -1.52)
  line L15 (-0.25, -1.52) -> (-0.25, -1.02)
  line L16 (-0.25, -1.02) -> (0.25, -1.52) construction
  line L17 (0.25, -1.02) -> (-0.25, -1.52) construction
  point P0 (0, 1.27)
  point P1 (0, -1.27)
  dimension "d9" = 2.54
  dimension "d10" = 2.54
  dimension "d11" = 0.5
  dimension "d12" = 0.5
  dimension "d13" = 0.5
  dimension "d14" = 0.5
  constraint horizontal L0
  constraint perpendicular L0 L1
  constraint parallel L0 L2
  constraint parallel L1 L3
  constraint coincident L4 A0.centre
  constraint coincident L5 A0.centre
  constraint coincident A0.centre origin
  constraint horizontal L6
  constraint perpendicular L6 L7
  constraint parallel L6 L8
  constraint parallel L7 L9
  constraint coincident L10 P0
  constraint coincident L11 P0
  constraint midpoint L0 P0
  constraint horizontal L12
  constraint perpendicular L12 L13
  constraint parallel L12 L14
  constraint parallel L13 L15
  constraint coincident L16 P1
  constraint coincident L17 P1
  constraint midpoint L2 P1
  measures "d9" distance of L1.end L2.end
  measures "d10" distance of L0.end L1.end
  measures "d11" distance of L7.end L8.end
  measures "d12" distance of L6.end L7.end
  measures "d13" distance of L13.end L14.end
  measures "d14" distance of L12.end L13.end
extrude "Extrude3" add sketch "Sketch3" along normal blind 7 contours L6 L7 L8 L9 | L12 L13 L14 L15

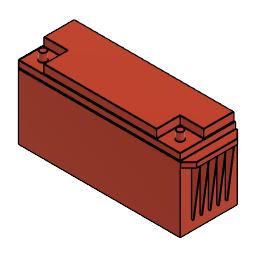
design "200ah_battery"
part number: 2026-09-24-16-06-27-907
Autodesk Fusion 360 part; units mm, degrees
sketch "Sketch1" plane through (0, 0, 0) normal (0, 0, 1) x (1, 0, 0)
  line L0 (-242.5, 85) -> (242.5, 85)
  line L1 (242.5, 85) -> (242.5, -85)
  line L2 (242.5, -85) -> (-242.5, -85)
  line L3 (-242.5, -85) -> (-242.5, 85)
  line L4 (-242.5, 85) -> (242.5, -85) construction
  line L5 (242.5, 85) -> (-242.5, -85) construction
  dimension "d1" = 485
  dimension "d2" = 170
  constraint horizontal L0
  constraint perpendicular L0 L1
  constraint parallel L0 L2
  constraint parallel L1 L3
  constraint coincident L4 origin
  constraint coincident L5 origin
  measures "d1" distance of L1.end L2.end
  measures "d2" distance of L0.end L1.end
extrude "Extrude1" add sketch "Sketch1" along normal blind 240
sketch "Sketch2" plane through (0, 0, 240) normal (0, 0, 1) x (-1, 0, 0)
  line L0 (242.5, 85) -> (-242.5, 85)
  line L1 (-242.5, 85) -> (-242.5, -85)
  line L2 (-242.5, -85) -> (242.5, -85)
  line L3 (242.5, -85) -> (242.5, 85)
  line L4 (-237.5, 80) -> (237.5, 80)
  line L5 (237.5, 80) -> (237.5, -80)
  line L6 (237.5, -80) -> (-237.5, -80)
  line L7 (-237.5, -80) -> (-237.5, 80)
  line L8 (-237.5, 80) -> (237.5, -80) construction
  line L9 (237.5, 80) -> (-237.5, -80) construction
  dimension "d5" = 475
  dimension "d6" = 160
  constraint horizontal L4
  constraint perpendicular L4 L5
  constraint parallel L4 L6
  constraint parallel L5 L7
  constraint coincident L8 origin
  constraint coincident L9 origin
  measures "d5" distance of L5.end L6.end
  measures "d6" distance of L4.end L5.end
extrude "Extrude2" cut sketch "Sketch2" against normal blind 25
sketch "Sketch3" plane through (0, 0, 240) normal (0, 0, 1) x (-1, 0, 0)
  line L0 (-237.5, 80) -> (-237.5, -80)
  line L1 (-237.5, -80) -> (237.5, -80)
  line L2 (237.5, -80) -> (237.5, 80)
  line L3 (237.5, 80) -> (-237.5, 80)
  line L4 (-237.5, 80) -> (-167.5, 80)
  line L5 (-167.5, 80) -> (-167.5, 10)
  line L6 (-167.5, 10) -> (-237.5, 10)
  line L7 (-237.5, 10) -> (-237.5, 80)
  line L8 (237.5, 80) -> (167.5, 80)
  line L9 (167.5, 80) -> (167.5, 10)
  line L10 (167.5, 10) -> (237.5, 10)
  line L11 (237.5, 10) -> (237.5, 80)
  dimension "d9" = 70
  dimension "d10" = 70
  dimension "d11" = 70
  dimension "d12" = 70
  constraint horizontal L4
  constraint vertical L5
  constraint horizontal L6
  constraint vertical L7
  constraint coincident L0.start L3.end
  constraint horizontal L8
  constraint vertical L9
  constraint horizontal L10
  constraint vertical L11
  constraint coincident L2.end L3.start
  measures "d9" distance of L0.start L4.end
  measures "d10" distance of L0.start L6.end
  measures "d11" distance of L2.end L8.end
  measures "d12" distance of L2.end L10.end
extrude "Extrude3" cut sketch "Sketch3" against normal blind 25 contours L0 L3 L4 L5 L6 L7 | L2 L3 L8 L9 L10 L11
sketch "Sketch4" plane through (0, 0, 215) normal (0, 0, 1) x (-1, 0, 0)
  line L0 (237.5, -80) -> (-237.5, -80)
  line L1 (-237.5, -80) -> (-237.5, 10)
  line L2 (-237.5, 10) -> (-167.5, 10)
  line L3 (-167.5, 10) -> (-167.5, 80)
  line L4 (-167.5, 80) -> (167.5, 80)
  line L5 (167.5, 80) -> (167.5, 10)
  line L6 (167.5, 10) -> (237.5, 10)
  line L7 (237.5, 10) -> (237.5, -80)
  line L8 (242.5, -85) -> (242.5, 85)
  line L9 (242.5, 85) -> (-242.5, 85)
  line L10 (-242.5, 85) -> (-242.5, -85)
  line L11 (-242.5, -85) -> (242.5, -85)
  line L12 (240, -82.5) -> (-240, -82.5)
  line L13 (-240, -82.5) -> (-240, 82.5)
  line L14 (-240, 82.5) -> (240, 82.5)
  line L15 (240, 82.5) -> (240, -82.5)
  line L16 (240, -82.5) -> (-240, 82.5) construction
  line L17 (-240, -82.5) -> (240, 82.5) construction
  dimension "d15" = 480
  dimension "d16" = 165
  constraint horizontal L12
  constraint perpendicular L12 L13
  constraint parallel L12 L14
  constraint parallel L13 L15
  constraint coincident L16 origin
  constraint coincident L17 origin
  measures "d15" distance of L13.end L14.end
  measures "d16" distance of L12.end L13.end
extrude "Extrude4" cut sketch "Sketch4" against normal blind 20 contours L8 L9 L10 L11
sketch "Sketch5" plane through (242.5, 0, 0) normal (1, 0, 0) x (0, 1, 0)
  line L0 (85, 195) -> (-85, 195)
  line L1 (-85, 195) -> (-85, 0)
  line L2 (-85, 0) -> (85, 0)
  line L3 (85, 0) -> (85, 195)
  line L4 (-85, 195) -> (85, 195)
  line L5 (85, 195) -> (85, 180)
  line L6 (85, 180) -> (-85, 180)
  line L7 (-85, 180) -> (-85, 195)
  dimension "d19" = 15
  constraint horizontal L4
  constraint vertical L5
  constraint horizontal L6
  constraint vertical L7
  constraint coincident L0.end L1.start
  measures "d19" distance of L0.end L6.end
extrude "Extrude5" add sketch "Sketch5" along normal blind 25 contours L0 L1 L3 L4 L5 L6 L7
sketch "Sketch6" plane through (-242.5, 0, 0) normal (-1, 0, 0) x (0, -1, 0)
  line L0 (85, 195) -> (-85, 195)
  line L1 (-85, 195) -> (-85, 0)
  line L2 (-85, 0) -> (85, 0)
  line L3 (85, 0) -> (85, 195)
  line L4 (-85, 195) -> (85, 195)
  line L5 (85, 195) -> (85, 180)
  line L6 (85, 180) -> (-85, 180)
  line L7 (-85, 180) -> (-85, 195)
  dimension "d22" = 15
  constraint horizontal L4
  constraint vertical L5
  constraint horizontal L6
  constraint vertical L7
  constraint coincident L0.end L1.start
  measures "d22" distance of L0.end L6.end
extrude "Extrude6" add sketch "Sketch6" along normal blind 20 contours L0 L1 L3 L4 L5 L6 L7
chamfer "Chamfer1" distance 24 angle 45 4 edges at (-262.5, 85, 187.5) (-262.5, -85, 187.5) (267.5, 85, 187.5) (267.5, -85, 187.5)
sketch "Sketch7" plane through (-242.5, 0, 0) normal (-1, 0, 0) x (0, -1, 0)
  line L0 (81, 0) -> (81, 180)
  line L1 (81, 180) -> (-81, 180)
  line L2 (-81, 180) -> (-81, 0)
  line L3 (-81, 0) -> (81, 0)
  line L4 (0, 180) -> (0, 30) construction
  line L5 (-1, 180) -> (1, 180)
  line L6 (1, 180) -> (1, 30)
  line L7 (1, 30) -> (-1, 30)
  line L8 (-1, 30) -> (-1, 180)
  line L9 (-1, 180) -> (1, 30) construction
  line L10 (1, 180) -> (-1, 30) construction
  point P0 (0, 105)
  dimension "d26" = 2
  constraint midpoint L1 L4.start
  constraint perpendicular L1 L4
  constraint horizontal L5
  constraint perpendicular L5 L6
  constraint parallel L5 L7
  constraint parallel L6 L8
  constraint coincident L9 P0
  constraint coincident L10 P0
  constraint midpoint L4 P0
  measures "d26" distance of L6.end L7.end
extrude "Extrude7" add sketch "Sketch7" along normal blind 20 contours L1 L5 L6 L7 L8
pattern_linear "R-Pattern2" count 1 spacing 0 along (0, 0, -1) count 5 spacing 25 along (0, 1, 0) both ways of "Extrude7"
extrude "Extrude8" add 1 faces at (-262.5, 0.3333, 190) along direction (1, 0, 0) blind 530
chamfer "Chamfer2" distance 150 distance2 20 14 edges at (-262.5, 50, 30) (-262.5, 25, 30) (-262.5, -50, 30) (-262.5, 0, 30) (-262.5, -50, 30) (-262.5, 0, 30) (-262.5, -25, 30) (267.5, 50, 30) (267.5, 25, 30) (267.5, 0, 30) (267.5, -50, 30) (267.5, -25, 30) (267.5, 0, 30) (267.5, -50, 30) measured on face at (-262.5, 0.3333, 190) measured on face at (-262.5, 0.3333, 190) measured on face at (-262.5, 0.3333, 190) measured on face at (-262.5, 0.3333, 190) measured on face at (-262.5, 0.3333, 190) measured on face at (-262.5, 0.3333, 190) measured on face at (-262.5, 0.3333, 190) measured on face at (267.5, -0.3333, 190) measured on face at (267.5, -0.3333, 190) measured on face at (267.5, -0.3333, 190) measured on face at (267.5, -0.3333, 190) measured on face at (267.5, -0.3333, 190) measured on face at (267.5, -0.3333, 190) measured on face at (267.5, -0.3333, 190)
sketch "Sketch8" plane through (0, 0, 215) normal (0, 0, 1) x (-1, 0, 0)
  line L0 (240, -82.5) -> (240, 82.5)
  line L1 (240, 82.5) -> (-240, 82.5)
  line L2 (-240, 82.5) -> (-240, -82.5)
  line L3 (-240, -82.5) -> (240, -82.5)
  line L4 (237.5, -80) -> (-237.5, -80)
  line L5 (-237.5, -80) -> (-237.5, 10)
  line L6 (-237.5, 10) -> (-167.5, 10)
  line L7 (-167.5, 10) -> (-167.5, 80)
  line L8 (-167.5, 80) -> (167.5, 80)
  line L9 (167.5, 80) -> (167.5, 10)
  line L10 (167.5, 10) -> (237.5, 10)
  line L11 (237.5, 10) -> (237.5, -80)
  line L12 (167.5, 10) -> (240, 82.5) construction
  line L13 (-167.5, 10) -> (-240, 82.5) construction
  circle A0 centre (-203.75, 46.25) radius 10
  circle A1 centre (203.75, 46.25) radius 10
  dimension "d41" = 20
  dimension "d42" = 20
  constraint coincident L9.end L10.start
  constraint coincident L0.end L1.start
  constraint coincident L6.end L7.start
  constraint coincident L1.end L2.start
  constraint midpoint L13 A0.centre
  constraint midpoint L12 A1.centre
  measures "d41" diameter of A0
  measures "d42" diameter of A1
extrude "Extrude9" add sketch "Sketch8" along normal blind 25 contours L4 L5 L6 L7 L8 L9 L10 L11 | A0 | A1
fillet "Fillet1" radius 1 2 edges at (-194.4267, -42.6338, 240) (213.0733, -42.6338, 240)
fillet "Fillet2" radius 1 1 faces at (-55.8333, 50, 240)
fillet "Fillet3" radius 1 1 faces at (-202.5149, -18.7743, 215)
fillet "Fillet4" radius 1 1 faces at (249.1667, 20.3333, 195)

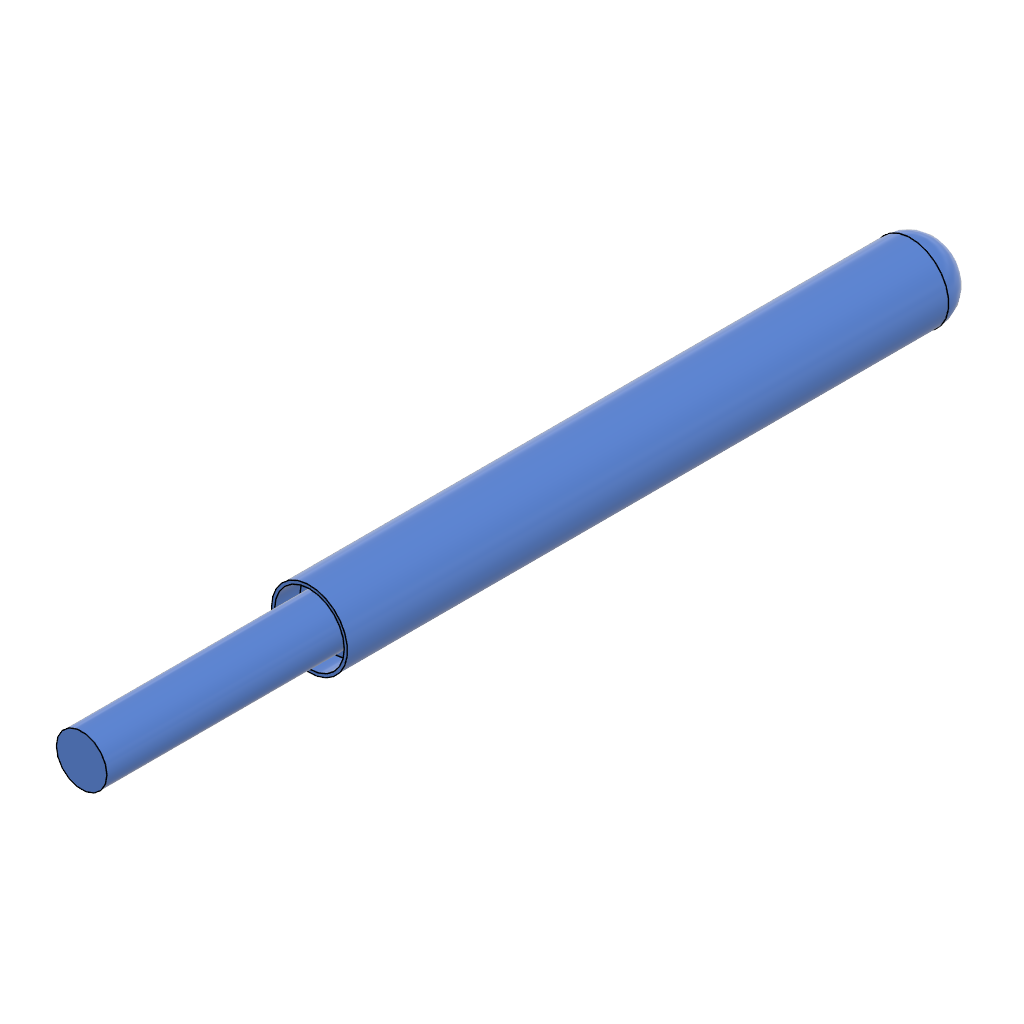
design "DS18B20"
part number: 2026-09-25-10-57-52-979
Autodesk Fusion 360 part; units mm, degrees
sketch "Sketch1" plane through (0, 0, 0) normal (0, 0, 1) x (1, 0, 0)
  circle A0 centre (0, 0) radius 3
  dimension "d1" = 6
  constraint coincident A0.centre origin
  measures "d1" diameter of A0
extrude "Extrude1" add sketch "Sketch1" along normal blind 50
fillet "Fillet1" radius 2.5 1 edges at (-2.797, -1.0848, 0)
sketch "Sketch2" plane through (0, 0, 50) normal (0, 0, 1) x (1, 0, 0)
  circle A0 centre (0, 0) radius 3
  circle A1 centre (0, 0) radius 2.75
  dimension "d6" = 5.5
  constraint concentric A0 A1
  measures "d6" diameter of A1
extrude "Extrude2" cut sketch "Sketch2" against normal blind 2 contours A1
sketch "Sketch3" plane through (0, 0, 48) normal (0, 0, 1) x (1, 0, 0)
  circle A0 centre (0, 0) radius 2.75
  circle A1 centre (0, 0) radius 2
  dimension "d9" = 4
  constraint coincident A0.centre A1.centre
  measures "d9" diameter of A1
extrude "Extrude3" add sketch "Sketch3" along normal blind 20 contours A1

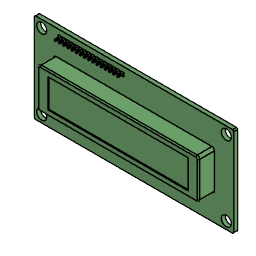
design "LCD_16X2"
part number: 2026-09-24-15-06-06-234
Autodesk Fusion 360 part; units mm, degrees
sketch "Sketch1" plane through (0, 0, 0) normal (0, 1, 0) x (1, 0, 0)
  line L0 (-40, -18) -> (40, -18)
  line L1 (40, -18) -> (40, 18)
  line L2 (40, 18) -> (-40, 18)
  line L3 (-40, 18) -> (-40, -18)
  line L4 (-40, -18) -> (40, 18) construction
  line L5 (40, -18) -> (-40, 18) construction
  dimension "d1" = 80
  dimension "d2" = 36
  constraint horizontal L0
  constraint perpendicular L0 L1
  constraint parallel L0 L2
  constraint parallel L1 L3
  constraint coincident L4 origin
  constraint coincident L5 origin
  measures "d1" distance of L1.end L2.end
  measures "d2" distance of L0.end L1.end
extrude "Extrude1" add sketch "Sketch1" along normal blind 1.6
sketch "Sketch2" plane through (0, 0, 0) normal (0, -1, 0) x (1, 0, 0)
  line L0 (-40, 18) -> (-40, -18)
  line L1 (-40, -18) -> (40, -18)
  line L2 (40, -18) -> (40, 18)
  line L3 (40, 18) -> (-40, 18)
  line L4 (32.25, 8) -> (-32.25, 8)
  line L5 (-32.25, 8) -> (-32.25, -8)
  line L6 (-32.25, -8) -> (32.25, -8)
  line L7 (32.25, -8) -> (32.25, 8)
  line L8 (32.25, 8) -> (-32.25, -8) construction
  line L9 (-32.25, 8) -> (32.25, -8) construction
  line L10 (-28.1, 5.75) -> (28.1, 5.75)
  line L11 (28.1, 5.75) -> (28.1, -5.75)
  line L12 (28.1, -5.75) -> (-28.1, -5.75)
  line L13 (-28.1, -5.75) -> (-28.1, 5.75)
  line L14 (-28.1, 5.75) -> (28.1, -5.75) construction
  line L15 (28.1, 5.75) -> (-28.1, -5.75) construction
  dimension "d5" = 64.5
  dimension "d6" = 16
  dimension "d7" = 56.2
  dimension "d8" = 11.5
  constraint horizontal L4
  constraint perpendicular L4 L5
  constraint parallel L4 L6
  constraint parallel L5 L7
  constraint coincident L8 origin
  constraint coincident L9 origin
  constraint horizontal L10
  constraint perpendicular L10 L11
  constraint parallel L10 L12
  constraint parallel L11 L13
  constraint coincident L14 origin
  constraint coincident L15 origin
  measures "d5" distance of L5.end L6.end
  measures "d6" distance of L4.end L5.end
  measures "d7" distance of L11.end L12.end
  measures "d8" distance of L10.end L11.end
extrude "Extrude2" add sketch "Sketch2" along normal blind 6.4 contours L4 L5 L6 L7
extrude "Extrude3" add 1 faces at (-9.3667, 0, 1.9167) along direction (0, -1, 0) blind 6